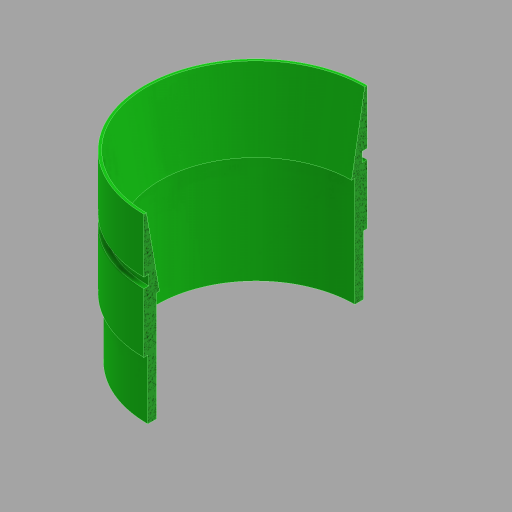
# Autodesk Inventor part: CapConeThin
Saved by Autodesk Inventor 2024 (Build 280153020, 153B)
## iProperties
Created: 2023-09-22
Part Number: CapConeThin
Material: Brass
Document SubType Name: Modeling
Designer: schanen
Density: 8.49 g/cm^3
Appearance: Dark Green
Author: schanen
Autodesk Inventor part; units mm, degrees
ref_plane "YZ Plane" through (0, 0, 0) normal (1, 0, 0) x (0, 1, 0)
ref_plane "XZ Plane" through (0, 0, 0) normal (0, 1, 0) x (-1, 0, 0)
ref_plane "XY Plane" through (0, 0, 0) normal (0, 0, 1) x (1, 0, 0)
sketch "Sketch1" plane through (0, 0, 0) normal (0, 0, 1) x (1, 0, 0)
  line L0 (-21.725, -10) -> (-22.225, -10) construction
  line L1 (-22.225, -10) -> (-22.225, 0) construction
  line L2 (-22.225, 0) -> (-21.725, 0) construction
  line L3 (-21.725, 0) -> (-21.725, -10) construction
  line L4 (-22, 37) -> (-19.3551, 22)
  line L5 (-22.5, 12) -> (-22.5, 24)
  line L6 (-22.5, 24) -> (-21.5, 24)
  line L7 (-21.5, 24) -> (-21.5, 26)
  line L8 (-21.5, 26) -> (-22.5, 26)
  line L9 (-22.5, 26) -> (-22.5, 37)
  line L10 (-22, 37) -> (-22.5, 37)
  line L11 (0, -19.4) -> (0, 46.4) projected
  line L12 (-20, 22) -> (-19.3551, 22)
  line L13 (-22.5, 12) -> (-21.725, 12)
  line L14 (-21.725, 12) -> (-21.725, 0)
  line L15 (-21.725, 0) -> (-20, 0)
  line L16 (-20, 0) -> (-20, 22)
  point P0 (0, 0)
  dimension "d0" = 10
  dimension "d1" = 22.225
  dimension "d3" = 0.5
  dimension "d5" = 11
  dimension "d6" = 2
  dimension "d7" = 22.5
  dimension "d12" = 1
  dimension "d18" = 0.5
  dimension "d19" = 10
  dimension "d20" = 15
  dimension "d21" = 12
  dimension "d22" = 37
  dimension "d24" = 20
  constraints: 32 end point, 6 perpendicular, 4 horizontal, 2 horizontal alignment, 2 parallel, 2 point on line, 2 vertical, 1 vertical alignment
  measures "d0" distance of L0.end L1.end
  measures "d1" distance from line of point (0, 0) L1
  measures "d3" distance of L0.end L0.start
  measures "d5" distance of L8.end L9.end
  measures "d6" distance of L6.end L7.end
  measures "d7" distance from line of point (0, 0) L5
  measures "d12" distance of L5.end L6.end
  measures "d18" distance of L4.start L9.end
  measures "d19" angle of L4 L9
  measures "d20" vertical distance of L9.end L12.start
  measures "d21" distance of L13.end L14.end
  measures "d22" vertical distance of L2.end L9.end
  measures "d24" distance from line of point (0, 0) L16
revolve "Revolution1" add sketch "Sketch1" angle 360 about axis through (0, -10, 0) along (0, 1, 0)
body "Solid1"
